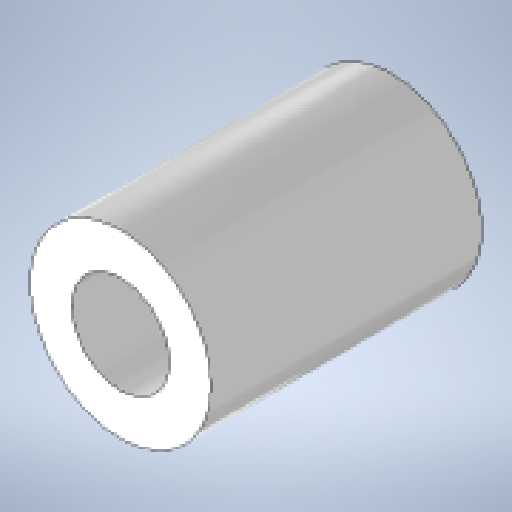
# Autodesk Inventor part: Wedge Mount
Saved by Autodesk Inventor 2023.2 (Build 272271000, 271)
## iProperties
Created: 2024-04-01
Part Number: Wedge Mount
Material: UHMW, White
Document SubType Name: Modeling
Designer: Nathan Cai
Density: 0.94 g/cm^3
Appearance: Smooth - White
Mass: 7.49207 g
Surface Area: 37.8303 cm^2
Volume: 7.97029 cm^3
Author: Nathan Cai
Autodesk Inventor part; units mm, degrees
ref_plane "YZ Plane" through (0, 0, 0) normal (1, 0, 0) x (0, 1, 0)
ref_plane "XZ Plane" through (0, 0, 0) normal (0, 1, 0) x (-1, 0, 0)
ref_plane "XY Plane" through (0, 0, 0) normal (0, 0, 1) x (1, 0, 0)
sketch "Sketch3" plane through (0, 0, 0) normal (0, 0, 1) x (1, 0, 0)
  circle A0 centre (0, 0) radius 3.429
  circle A1 centre (0, 0) radius 6.35
  line L0 (6.35, 22.225) -> (-19.1908, 0.7937)
  line L1 (-19.1908, 0.7937) -> (-6.3002, 0.7937)
  line L2 (6.35, 22.225) -> (6.35, 0)
  dimension "d23" = 6.858
  dimension "d24" = 12.7
  dimension "d27" = 0.7937
  dimension "d28" = 6.35
  dimension "d29" = 50
  dimension "d30" = 22.225
  constraints: 6 end point, 2 centre point, 2 coincident, 2 point on circle, 1 horizontal, 1 perpendicular
  measures "d23" diameter of A0
  measures "d24" diameter of A1
  measures "d27" distance from line of point (0, 0) L1
  measures "d28" distance from line of L2 point (0, 0)
  measures "d29" angle of L2 L0
  measures "d30" vertical distance of point (0, 0) L0.start
extrude "Extrusion3" add sketch "Sketch3" along normal blind 19.05
fillet "Fillet2" radius 6.35 1 edges at (-6.3002, 0.7938, 9.525)
sketch "Sketch4" plane through (-19.1908, 0.7938, 19.05) normal (-0.6427876, 0.7660444, 0) x (0.7660444, 0.6427876, 0)
  line L0 (33.3411, 0) -> (0, 0) projected
  line L1 (6.35, 0) -> (6.35, 18.8766) construction
  line L2 (0, 19.05) -> (0, 0) projected
  line L3 (0, 9.525) -> (33.3411, 9.525) construction
  line L4 (33.3411, 19.05) -> (33.3411, 0) projected
  point P0 (14.1908, 19.05)
  point P1 (6.35, 3.175)
  point P2 (6.35, 15.875)
  point P3 (16.1742, 15.875)
  point P4 (16.1742, 3.175)
  point P5 (25.9983, 15.875)
  point P6 (25.9983, 3.175)
  dimension "d33" = 6.35
  dimension "d34" = 3.175
  dimension "d45" = 9.8242
  constraints: 4 end point, 2 midpoint, 2 point on line, 1 horizontal, 1 symmetric about line, 1 vertical, 4 other
  measures "d33" distance between parallel lines of L2 L1
  measures "d34" distance from line of L0 point (6.35, 3.175)
  measures "d45" distance of point (6.35, 15.875) point (16.174, 15.875)
hole "Hole1" at (-14.3264, 4.8755, 15.875) at (-14.3264, 4.8755, 3.175) at (-6.8006, 11.1903, 15.875) at (-6.8006, 11.1903, 3.175) at (0.7251, 17.5052, 3.175) at (0.7251, 17.5052, 15.875) direction (0.6427876, -0.7660444, 0) diameter 2.54 depth 6.35 tip angle 118
fillet "Fillet4" radius 1.5875 2 edges at (-19.1908, 0.7937, 9.525) (6.35, 22.225, 9.525)
body "Solid2"
